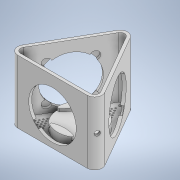
# Autodesk Inventor part: Reactor small aircooled
Saved by Autodesk Inventor 2022.4 (Build 264492010, 492A)
## iProperties
Created: 2023-03-20
Part Number: Reactor small aircooled
Material: Generic
Document SubType Name: Modeling
Designer: tmass
Density: 1 g/cm^3
Appearance: Default
Author: tmass
Autodesk Inventor part; units mm, degrees
ref_plane "YZ Plane" through (0, 0, 0) normal (1, 0, 0) x (0, 1, 0)
sketch "Sketch1" plane through (0, 0, 0) normal (0, 1, 0) x (-1, 0, 0)
  line L0 (46.7654, 37) -> (-46.7654, 37)
  line L1 (-55.4256, 22) -> (-8.6603, -59)
  line L2 (8.6603, -59) -> (55.4256, 22)
  line L3 (0, -169.4892) -> (0, 106.9349) construction
  line L4 (106.385, 61.4214) -> (0, 0) construction
  line L5 (0, 0) -> (-106.3874, 61.4228) construction
  line L6 (0, 0) -> (0, -130) construction
  arc A0 (-46.7654, 37) -> (-55.4256, 22) centre (-46.7654, 27) ccw
  arc A1 (-8.6603, -59) -> (8.6603, -59) centre (0, -54) ccw
  arc A2 (55.4256, 22) -> (46.7654, 37) centre (46.7654, 27) ccw
  point P0 (64.0859, 37)
  point P1 (0, -74)
  point P2 (-64.0859, 37)
  point P3 (64.0859, 37)
  point P4 (-64.0859, 37)
  point P5 (0, -74)
  point P6 (0, -74)
  point P7 (64.0859, 37)
  point P8 (-64.0859, 37)
  dimension "d19" = 0
  dimension "d21" = 0
  dimension "d4" = 37
  dimension "d5" = 37
  dimension "d6" = 37
  dimension "d12" = 30
  dimension "d13" = 30
  dimension "d14" = 30
  dimension "d15" = 30
  dimension "d16" = 30
  dimension "d17" = 30
  dimension "d18" = 212.7724
  dimension "d36" = 120
  dimension "d37" = 120
  dimension "d38" = 120
  dimension "d132" = 10
  dimension "d133" = 10
  constraints: 12 end point, 10 point on line, 6 point on circle, 6 tangent, 3 centre point, 2 horizontal, 1 equal radius, 15 other
  measures "d4" distance from line of L0 L4.end
  measures "d5" distance from line of L4.end L1
  measures "d6" distance from line of L4.end L2
  measures "d12" angle of L1 L3
  measures "d13" angle of L2 L3
  measures "d14" angle of L4 L2
  measures "d15" angle of L0 L4
  measures "d16" angle of L0 L5
  measures "d17" angle of L1 L5
  measures "d18" distance of L4.start L5.end
  measures "d36" angle of L4 L3
  measures "d37" angle of L5 L4
  measures "d38" angle of L3 L5
  measures "d132" radius of A0
  measures "d133" radius of A1
extrude "Extrusion1" add sketch "Sketch1" along normal blind 85
shell "Shell1" thickness 4 removed faces 1 at (2.8868, 85, 5)
sketch "Sketch16" plane through (0, 0, -74) normal (0.8660254, 0, -0.5) x (-0.5, 0, -0.8660254)
  circle A0 centre (-64.0859, 38.75) radius 32
  line L0 (-64.0859, 0) -> (-64.0859, 108.3502)
  line L1 (0, 0) -> (0, 100) projected
  line L2 (-110.8513, 0) -> (-17.3205, 0) projected
  dimension "d113" = 64
  dimension "d130" = 64.0859
  dimension "d149" = 38.75
  constraints: 2 end point, 1 centre point, 1 point on line, 1 vertical
  measures "d113" diameter of A0
  measures "d130" distance between parallel lines of L1 L0
  measures "d149" distance from line of A0.centre L2
extrude "Extrusion9" cut sketch "Sketch16" against normal blind 5
sketch "Sketch4" plane through (0, 0, -74) normal (0.8660254, 0, -0.5) x (-0.5, 0, -0.8660254)
  circle A0 centre (-64.0859, 38.75) radius 32 projected
  circle A1 centre (-64.0859, 38.75) radius 32
  circle A2 centre (-64.0859, 38.75) radius 37
  circle A3 centre (-88.0859, 62.75) radius 5.5
  line L0 (-163.3275, 38.75) -> (-64.0859, 38.75) construction
  line L1 (-64.0859, 111.6616) -> (-64.0859, -27.0146) construction
  line L2 (-88.0859, 62.75) -> (-64.0859, 38.75)
  circle A4 centre (-88.0859, 14.75) radius 5.5
  circle A5 centre (-40.0859, 14.75) radius 5.5
  circle A6 centre (-40.0859, 62.75) radius 5.5
  line L3 (-110.8513, 0) -> (-17.3205, 0) projected
  circle A7 centre (-64.0859, 38.75) radius 32 projected
  point P0 (-64.0859, 0)
  point P1 (-64.0859, 0)
  point P2 (-128.1718, 0)
  point P3 (0, 0)
  point P4 (-32.0859, 38.75)
  point P5 (-32.0859, 38.75)
  dimension "d30" = 74
  dimension "d39" = 45
  dimension "d40" = 24
  dimension "d41" = 11
  dimension "d44" = 360
  constraints: 6 centre point, 6 end point, 4 coincident, 4 point on line, 2 concentric, 1 horizontal, 1 midpoint, 1 perpendicular, 1 vertical, 11 other
  measures "d30" diameter of A2
  measures "d39" angle of L2 L0
  measures "d40" horizontal distance of A0.centre L2.start
  measures "d41" diameter of A3
ref_plane "Work Plane1" through (32.1695, 9, 5) normal (0, 1, 0) x (1, 0, 0)
sketch "Sketch8" plane through (32.1695, 9, 5) normal (0, 1, 0) x (1, 0, 0)
  circle A0 centre (-32.1695, 5) radius 30
  line L0 (10, 10) -> (10, 5.9602) projected
  point P0 (-32.1695, 5)
  point P1 (10, 0)
  dimension "d131" = 60
  constraints: 1 centre point, 1 coincident
  measures "d131" diameter of A0
extrude "Extrusion6" add sketch "Sketch8" along normal blind 2 and the other way blind 6.25
sketch "Sketch11" plane through (0, 0, 0) normal (0, 0, 1) x (1, 0, 0)
  point P0 (0, 0)
sketch "Sketch12" plane through (51.0955, 4, 22.5) normal (-0.8660254, 0, 0.5) x (0.5, 0, 0.8660254)
  circle A0 centre (-69.0333, 10.75) radius 5.5 projected
  circle A1 centre (-62.3538, 56) radius 32 projected
  circle A2 centre (-69.0333, 58.75) radius 5.5 projected
  circle A3 centre (-21.0333, 58.75) radius 5.5 projected
  circle A4 centre (-21.0333, 10.75) radius 5.5 projected
  circle A5 centre (-45.0333, 34.75) radius 32 projected
  circle A6 centre (-21.0333, 10.75) radius 5.5
  circle A7 centre (-69.0333, 10.75) radius 5.5
  circle A8 centre (-69.0333, 58.75) radius 5.5
  circle A9 centre (-21.0333, 58.75) radius 5.5
  point P0 (-45.0333, -4)
  constraints: 4 centre point, 4 coincident, 4 concentric
extrude "Extrusion8" cut sketch "Sketch12" against normal blind 3.5 contours A0 A5 | A5 A0 | A5 A4 | A4 A5 | A5 A2 | A2 A5 | A5 A3 | A3 A5
pattern_circular "Circular Pattern3" count 3 over 360 about axis through (0, -10, 0) along (0, 1, 0) of "Extrusion8", "Extrusion9"
pattern_circular "Circular Pattern4" count 3 over 360 about axis through (0, -10, 0) along (0, 1, 0) of "Extrusion9", "Extrusion8"
sketch "Sketch19" plane through (32.1695, 11, 5) normal (0, 1, 0) x (1, 0, 0)
  circle A0 centre (-88.3365, 37.428) radius 44.5
  line L0 (-88.3365, 37.428) -> (-32.1695, 5)
  line L1 (-40.8298, 64) -> (-87.5952, -17) projected
  circle A1 centre (23.9974, 37.428) radius 44.5
  line L2 (-32.1695, 5) -> (23.9974, 37.428)
  line L3 (23.2561, -17) -> (-23.5093, 64) projected
  circle A2 centre (-32.1695, -59.856) radius 44.5
  line L4 (-32.1695, 5) -> (-32.1695, -59.856)
  circle A3 centre (-32.1695, 5) radius 30
  point P0 (39.9953, 0)
  point P1 (-14.3036, -19.0999)
  point P2 (-50.0355, -19.0999)
  point P3 (-20.2314, 32.5224)
  point P4 (-2.3654, 1.5776)
  point P5 (-61.9737, 1.5776)
  point P6 (-44.1077, 32.5224)
  dimension "d140" = 64.856
  dimension "d141" = 89
  dimension "d142" = 89
  dimension "d143" = 64.856
  dimension "d144" = 89
  dimension "d145" = 64.856
  constraints: 6 end point, 4 centre point, 2 perpendicular, 1 coincident, 1 vertical
  measures "d140" distance of L0.start L0.end
  measures "d141" diameter of A0
  measures "d142" diameter of A1
  measures "d143" distance of L0.end L2.end
  measures "d144" diameter of A2
  measures "d145" distance of L0.end L4.end
extrude "Extrusion10" add sketch "Sketch19" along normal blind 4 contours A0 L0 A3 | A0 A3 L0 | A3 L2 A1 | L2 A3 A1 | A2 L4 A3 | A2 A3 L4
sketch "Sketch20" plane through (0, 0, 0) normal (0, 0, 1) x (1, 0, 0)
  line L0 (-17.866, 11) -> (17.866, 11) projected
  line L1 (17.866, 11) -> (-17.866, 11)
  line L2 (-17.866, 11) -> (-17.866, 66.5)
  line L3 (-17.866, 66.5) -> (17.866, 66.5)
  line L4 (17.866, 66.5) -> (17.866, 11)
  line L5 (17.866, 66.5) -> (-17.866, 11)
  line L6 (-17.866, 66.5) -> (17.866, 11)
  line L7 (0, -54.7499) -> (0, 139.3969) projected
  line L8 (30, 0) -> (-30, 0) projected
  point P0 (0, 0)
  point P1 (0, 38.75)
  point P2 (0, 38.75)
  dimension "d148" = 55.5
  dimension "d150" = 38.75
  constraints: 12 end point, 2 midpoint, 2 parallel, 1 horizontal, 1 perpendicular, 1 point on line
  measures "d148" distance of L1.end L2.end
  measures "d150" distance from line of L8 point (0, 38.75)
sketch "Sketch21" plane through (0, 0, 0) normal (0, 0, 1) x (1, 0, 0)
  line L0 (30, 9) -> (21.2132, 9) projected
  line L1 (0, 0) -> (30, 9)
  line L2 (30, 9) -> (0, 9)
  line L3 (0, 9) -> (0, 0)
  line L4 (0, -54.7499) -> (0, 139.3969) projected
  constraints: 6 end point, 1 collinear, 1 perpendicular
revolve "Revolution4" add sketch "Sketch21" angle 360 about axis through (0, -10, 0) along (0, 1, 0)
fillet "Fillet1" radius 2 6 edges at (-29.8041, 13, 3.4224) (-11.9382, 13, -27.5224) (11.9382, 13, -27.5224) (-17.866, 13, 24.0999) (17.866, 13, 24.0999) (29.8041, 13, 3.4224)
ref_plane "Work Plane2" through (46.7654, 0, 37) normal (-0.8660254, 0, -0.5) x (0, 1, 0)
sketch "Sketch24" plane through (46.7654, 0, 37) normal (-0.8660254, 0, -0.5) x (0, 1, 0)
  line L0 (0, 0) -> (85, 0) projected
  line L1 (0, 17.3205) -> (85, 17.3205) projected
  line L2 (42.5, 0) -> (42.5, 17.3205)
  line L3 (0, 8.6603) -> (85, 8.6603)
  line L4 (85, 13.8564) -> (85, 3.4641) projected
  line L5 (0, 55.4256) -> (0, -38.1051) projected
  line L6 (85, 3.4641) -> (85, -43.3013) projected
  circle A0 centre (42.5, 8.6603) radius 3.25
  dimension "d193" = 42.5
  dimension "d194" = 42.5
  dimension "d195" = 85
  dimension "d196" = 6.5
  constraints: 4 end point, 3 midpoint, 1 centre point, 1 horizontal, 1 perpendicular
  measures "d193" distance between parallel lines of L4 L2
  measures "d194" distance between parallel lines of L5 L2
  measures "d195" distance between parallel lines of L5 L6
  measures "d196" diameter of A0
extrude "Extrusion12" cut sketch "Sketch24" against normal through all contours A0 L3 L2 | L2 L3 A0 | A0 L2 L3 | L2 A0 L3
sketch "Sketch25" plane through (-46.7654, 4, 33) normal (0, 1, 0) x (1, 0, 0)
  circle A0 centre (21.1962, 9) radius 1
  circle A1 centre (13.1962, 9) radius 1
  circle A2 centre (9.1962, 9) radius 1
  circle A3 centre (5.1962, 9) radius 1
  circle A4 centre (19.1962, 12.4641) radius 1
  circle A5 centre (17.1962, 15.9282) radius 1
  circle A6 centre (17.1962, 9) radius 1
  circle A7 centre (11.1962, 19.3923) radius 1
  circle A8 centre (9.1962, 15.9282) radius 1
  circle A9 centre (13.1962, 22.8564) radius 1
  circle A10 centre (7.1962, 12.4641) radius 1
  line L0 (21.1962, 9) -> (5.1962, 9)
  line L1 (5.1962, 9) -> (13.1962, 22.8564)
  line L2 (13.1962, 22.8564) -> (21.1962, 9)
  line L3 (93.5307, 0) -> (0, 0) projected
  line L4 (-5.1962, 9) -> (41.5692, 90) projected
  circle A11 centre (15.1962, 19.3923) radius 1
  line L5 (17.1962, 9) -> (11.1962, 19.3923)
  line L6 (9.1962, 15.9282) -> (13.1962, 9)
  line L7 (9.1962, 9) -> (7.1962, 12.4641)
  line L8 (19.1962, 12.4641) -> (7.1962, 12.4641)
  line L9 (17.1962, 15.9282) -> (9.1962, 15.9282)
  circle A12 centre (15.1962, 12.4641) radius 1
  circle A13 centre (13.1962, 15.9282) radius 1
  circle A14 centre (11.1962, 12.4641) radius 1
  point P0 (46.7654, 33)
  dimension "d201" = 60
  dimension "d202" = 60
  dimension "d203" = 9
  dimension "d204" = 9
  dimension "d205" = 2
  dimension "d206" = 2
  dimension "d207" = 2
  dimension "d208" = 2
  dimension "d209" = 2
  dimension "d210" = 2
  dimension "d211" = 2
  dimension "d212" = 2
  dimension "d213" = 2
  dimension "d214" = 2
  dimension "d215" = 2
  dimension "d216" = 4
  dimension "d217" = 4
  dimension "d218" = 4
  dimension "d219" = 4
  dimension "d220" = 4
  dimension "d221" = 4
  dimension "d222" = 4
  dimension "d223" = 4
  dimension "d224" = 4
  dimension "d225" = 2
  dimension "d227" = 4
  dimension "d228" = 2
  dimension "d229" = 2
  dimension "d230" = 2
  constraints: 16 end point, 15 centre point, 9 point on line, 7 midpoint, 1 horizontal
  measures "d201" angle of L0 L2
  measures "d202" angle of L1 L0
  measures "d203" distance from line of L0.start L3
  measures "d204" distance from line of L4 L1.end
  measures "d205" diameter of A0
  measures "d206" diameter of A1
  measures "d207" diameter of A2
  measures "d208" diameter of A3
  measures "d209" diameter of A10
  measures "d210" diameter of A4
  measures "d211" diameter of A5
  measures "d212" diameter of A7
  measures "d213" diameter of A6
  measures "d214" diameter of A8
  measures "d215" diameter of A9
  measures "d216" distance of L5.end L1.end
  measures "d217" distance of L6.start L5.end
  measures "d218" distance of L7.end L6.start
  measures "d219" distance of L0.end L7.end
  measures "d220" distance of L0.end L7.start
  measures "d221" distance of L7.start A1.centre
  measures "d222" distance of L5.start L6.end
  measures "d223" distance of L0.start L8.start
  measures "d224" distance of L8.start A5.centre
  measures "d225" diameter of A11
  measures "d227" distance of L9.start A11.centre
  measures "d228" diameter of A12
  measures "d229" diameter of A13
  measures "d230" diameter of A14
extrude "Extrusion13" cut sketch "Sketch25" against normal through all contours A0 L0 L2 | L2 L0 A0 | L2 A4 | A4 L8 L2 | L0 L5 A6 | A6 L0 | A4 L2 L8 | L5 L0 A6 | A12 L5 L8 | L8 L5 A12 | A12 L8 L5 | L0 L6 A1 | A1 L0 | L2 A5 | A5 L9 L2 | L8 A12 L5 | L6 L0 A1 | A5 L2 L9 | A13 L9 L5 | L5 L9 A13 | A14 L6 L8 | L8 L6 A14 | A14 L8 L6 | L0 L7 A2 | A2 L0 | L9 L5 A13 | L9 A13 L5 | L8 A14 L6 | L7 L0 A2 | A11 L2 | L2 A11 | L9 L1 A8 | A8 L6 L9 | A8 L1 L6 | L8 L1 A10 | A10 L7 L8 | A10 L1 L7 | L0 L1 A3 | A3 L1 L0 | L5 L1 A7 | A7 L1 L5 | L1 A8 | L1 A10 | L2 L1 A9 | A9 L1 L2 | A7 L1
sketch "Sketch26" plane through (-46.7654, 4, 33) normal (0, 1, 0) x (1, 0, 0)
  circle A0 centre (46.7654, 33) radius 30
  arc A1 (93.5307, -4) -> (102.191, 11) centre (93.5307, 6) ccw
  line L0 (0, -4) -> (93.5307, -4)
  arc A2 (-8.6603, 11) -> (0, -4) centre (0, 6) ccw
  line L1 (38.1051, 92) -> (-8.6603, 11)
  arc A3 (55.4256, 92) -> (38.1051, 92) centre (46.7654, 87) ccw
  line L2 (102.191, 11) -> (55.4256, 92)
  point P0 (46.7654, 33)
  point P1 (46.7654, 33)
  constraints: 6 end point, 6 point on circle, 4 centre point, 3 coincident
hole "Hole3" at (-46.7654, 4, 27) at (46.7654, 4, 27) at (0, 4, -54) direction (0, -1, 0) diameter 3.7 end through all
pattern_circular "Circular Pattern7" count 3 over 360 about axis through (0, -10, 0) along (0, 1, 0) of "Extrusion13"
equation "\"d5\" = d4"
equation "\"d6\" = d4"
body "Solid1"
